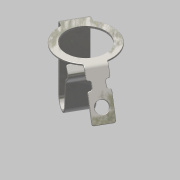
# Autodesk Inventor part: InputJack_signal2
Saved by Autodesk Inventor 2015 SP1 (Build 190203100, 203)
## iProperties
Created: 2015-06-13
Part Number: InputJack_signal2
Material: Generic
Document SubType Name: Modeling
Designer: Peter Mulkers
Density: 1 g/cm^3
Appearance: Titanium
Author: Peter Mulkers
Autodesk Inventor part; units mm, degrees
ref_plane "YZ Plane" through (0, 0, 0) normal (1, 0, 0) x (0, 1, 0)
ref_plane "XZ Plane" through (0, 0, 0) normal (0, 1, 0) x (-1, 0, 0)
ref_plane "XY Plane" through (0, 0, 0) normal (0, 0, 1) x (1, 0, 0)
sketch "Sketch1" plane through (0, 0, 0) normal (0, 0, 1) x (1, 0, 0)
  circle A0 centre (0, 0) radius 5.5
  line L0 (-6.9282, 4) -> (6.4952, -3.75) construction
  line L1 (0, 7.5) -> (0, -7.5) construction
  line L2 (-8.5532, 1.1854) -> (-5.3032, 6.8146)
  line L3 (-8.5532, 1.1854) -> (-7.4787, 0.565)
  line L4 (-5.3032, 6.8146) -> (-4.2287, 6.1942)
  line L5 (7.7452, -1.5849) -> (5.2452, -5.9151)
  line L6 (7.7452, -1.5849) -> (7.3737, -1.3705)
  line L7 (5.2452, -5.9151) -> (4.8737, -5.7006)
  arc A1 (-7.4787, 0.565) -> (4.8737, -5.7006) centre (0, 0) ccw
  arc A2 (7.3737, -1.3705) -> (-4.2287, 6.1942) centre (0, 0) ccw
  dimension "d0" = 11
  dimension "d2" = 60
  dimension "d3" = 6.5
  dimension "d4" = 8
  dimension "d5" = 15
  dimension "d6" = 5
  dimension "d7" = 7.5
  dimension "d8" = 7.5
  dimension "d9" = 7.5
  dimension "d10" = 2.5
  constraints: 16 end point, 7 point on circle, 4 perpendicular, 3 centre point, 3 midpoint, 2 coincident, 2 parallel, 1 point on line, 1 vertical alignment
  measures "d0" diameter of A0
  measures "d2" angle of L1 L0
  measures "d3" distance of L2.start L2.end
  measures "d4" distance from line of point (0, 0) L2
  measures "d5" distance of L1.start L1.end
  measures "d6" distance of L5.start L5.end
  measures "d7" radius of A2
  measures "d8" radius of A1
  measures "d9" distance from line of L5 A0.centre
  measures "d10" distance between parallel lines of L6 L0
extrude "Extrusion1" add sketch "Sketch1" along normal blind 0.5
sketch "Sketch2" plane through (5.6202, -6.1316, -0.25) normal (0.75, -0.4330127, 0.5) x (0.5, 0.8660254, 0)
  line L0 (5, 0) -> (0, 0)
  line L1 (0, 0) -> (0, -11.4226)
  line L2 (0, -11.4226) -> (5, -11.4226)
  line L3 (5, -11.4226) -> (5, 0)
  constraints: 8 end point
edge flange "Flange1" height 12 angle 60 thickness 0.5 bend radius 0.5 thickness toward (0.75, -0.4330127, 0.5) relief tear relief width 0.5 relief depth 0.25 edges at (6.4952, -3.75, 0) wall of the first edge with corners at (8.1202, -1.8014, -0.25) (5.6202, -6.1316, -0.25) (10.5663, -8.9872, -10.1423) (13.0663, -4.6571, -10.1423)
bend "Bend1"
corner "Corner1"
sketch "Sketch3" plane through (10.9413, -9.2037, -9.8923) normal (0.75, -0.4330127, 0.5) x (0.4330127, -0.25, -0.8660254)
  line L0 (-11.4226, 5) -> (-11.4226, 0) construction
  line L1 (0, 0) -> (-11.4226, 0) construction
  line L2 (0, 5) -> (0, 0) construction
  line L3 (-11.4226, 5) -> (0, 5) construction
  line L4 (-9, 0) -> (-9, 1)
  line L5 (-9, 1) -> (-7, 1)
  line L6 (-7, 1) -> (-7, 0)
  line L7 (-7, 0) -> (-9, 0)
  line L8 (-9, 5) -> (-9, 4)
  line L9 (-9, 4) -> (-7, 4)
  line L10 (-7, 4) -> (-7, 5)
  line L11 (-9, 5) -> (-7, 5)
  point P0 (-15.6057, 2.5)
  dimension "d23" = 1
  dimension "d25" = 2
  dimension "d26" = 7
  dimension "d27" = 1
  dimension "d28" = 2
  dimension "d29" = 7
  constraints: 16 end point, 4 perpendicular, 4 point on line, 2 collinear, 2 vertical
  measures "d23" distance between parallel lines of L5 L1
  measures "d25" distance between parallel lines of L6 L4
  measures "d26" distance between parallel lines of L2 L6
  measures "d27" distance between parallel lines of L3 L9
  measures "d28" distance between parallel lines of L10 L8
  measures "d29" distance between parallel lines of L2 L10
extrude "Extrusion2" cut sketch "Sketch3" against normal blind 0.5
fillet "Fillet1" radius 0.5 10 edges at (7.7228, -7.3455, -3.9551) (6.8567, -6.8455, -2.2231) (10.2228, -3.0154, -3.9551) (9.3567, -2.5154, -2.2231) (7.3567, -5.9795, -2.2231) (8.2228, -6.4795, -3.9551) (9.7228, -3.8814, -3.9551) (8.8567, -3.3814, -2.2231) (13.2538, -4.7654, -10.0173) (10.7538, -9.0955, -10.0173)
sketch "Sketch4" plane through (10.6268, -3.2486, -4.2631) normal (0.75, -0.4330127, 0.5) x (0.4330127, -0.25, -0.8660254)
  circle A0 centre (3, -2.5) radius 1.5
  line L0 (6.5, -0.5) -> (6.5, -4.5) projected
  point P0 (-9.1057, -2.5)
  point P1 (6.5, -2.5)
  dimension "d33" = 3
  dimension "d34" = 3.5
  constraints: 1 centre point, 1 horizontal alignment, 1 midpoint
  measures "d33" diameter of A0
  measures "d34" distance from line of A0.centre L0
extrude "Extrusion3" cut sketch "Sketch4" against normal blind 0.5
sketch "Sketch5" plane through (-5.7362, 7.0646, -0.5) normal (-0.8660254, 0.5, 0) x (-0.5, -0.8660254, 0)
  line L0 (6.5, 0) -> (0, 0)
  line L1 (0, 0) -> (0, -17)
  line L2 (0, -17) -> (6.5, -17)
  line L3 (6.5, -17) -> (6.5, 0)
  constraints: 6 end point, 1 horizontal, 1 perpendicular, 1 vertical
edge flange "Flange2" height 18 angle 90 thickness 0.5 bend radius 0.5 thickness toward (-0.8660254, 0.5, 0) relief tear relief width 0.5 relief depth 0.25 edges at (-6.9282, 4, 0) wall of the first edge with corners at (-8.9862, 1.4354, -0.5) (-5.7362, 7.0646, -0.5) (-5.7362, 7.0646, -17.5) (-8.9862, 1.4354, -17.5)
bend "Bend2"
corner "Corner2"
sketch "Sketch6" plane through (-9.4192, 1.6854, -17.5) normal (-0.5, -0.8660254, 0) x (0.8660254, -0.5, 0)
  line L0 (0, 17) -> (0, 0) construction
  arc A0 (0, 0) -> (4.9902, -0.2217) centre (2.5, 0) ccw
  line L1 (16.0711, 18) -> (2.2407, 18)
  line L2 (6, 10.5) -> (6, 7.5) construction
  line L3 (6, 9) -> (7.0607, 10.0607) construction
  line L4 (6, 9) -> (7.0607, 7.9393) construction
  line L5 (7.0607, 7.9393) -> (5.8421, 6.7208)
  line L6 (7.0607, 10.0607) -> (6, 11.1213)
  line L7 (4.9902, -0.2217) -> (5.5532, 6.1024)
  arc A1 (7.0607, 7.9393) -> (7.0607, 10.0607) centre (6, 9) ccw
  arc A2 (5.8421, 6.7208) -> (5.5532, 6.1024) centre (6.5492, 6.0137) ccw
  point P0 (9, 17.5)
  dimension "d47" = 5
  dimension "d48" = 9
  dimension "d50" = 6
  dimension "d51" = 45
  dimension "d52" = 45
  dimension "d53" = 1
  dimension "d54" = 1.5
  dimension "d55" = 1.5
  dimension "d56" = 1.7233
  dimension "d57" = 7.5
  dimension "d58" = 10.5
  measures "d47" diameter of A0
  measures "d48" distance from line of L1 L3.start
  measures "d50" distance from line of L0 L3.start
  measures "d51" angle of L3 L2
  measures "d52" angle of L4 L2
  measures "d53" radius of A2
  measures "d54" radius of A1
  measures "d55" distance of L3.end L6.end
  measures "d56" distance of L4.end L5.end
  measures "d57" distance from line of L2.start L1
  measures "d58" distance from line of L2.end L1
contour flange "Contour Flange1" sketch "Sketch6" thickness 0.5 bend radius 0.5 curves A0 L7 A2 L5 A1 L6 edges at (-7.3612, 4.25, -17.5) running between points at (-8.9862, 1.4354, -17.5) (-5.7362, 7.0646, -17.5)
bend "Bend3"
corner "Corner3"
fillet "Corner Round1" radius 0.5 6 edges at (-4.3762, -1.2262, -6.5555) (-1.1262, 4.403, -6.5555) (-7.4787, 0.565, 0.25) (-4.2287, 6.1942, 0.25) (4.8737, -5.7006, 0.25) (7.3737, -1.3705, 0.25)
fillet "Fillet2" radius 0.15 94 edges at (-7.5575, 0.528, 0.5) (-3.4091, -6.6804, 0.5) (4.8878, -5.8074, 0.5) (7.4733, -1.3293, 0.5) (4.0809, 6.2926, 0.5) (-4.236, 6.281, 0.5) (-9.1656, 1.539, 0.2071) (-9.4192, 1.6854, -9) (-7.3503, 0.4909, -19.9975) (-4.8538, -0.9504, -14.5597) (-4.532, -1.1362, -11.063) (-3.8322, -1.5403, -10.1699) (-2.924, -2.0646, -8.5) (-3.6107, -1.6681, -7.0858) (-4.0602, -1.2395, -6.4822) (-2.5981, 1.5, -6.3787) (-0.9566, 4.136, -6.4822) (-0.3607, 3.961, -7.0858) (0.326, 3.5646, -8.5) (-0.5822, 4.0889, -10.1699) (-1.282, 4.493, -11.063) (-1.6038, 4.6788, -14.5597) (-4.1003, 6.1201, -19.9975) (-6.1692, 7.3146, -9) (-5.9156, 7.1681, 0.2071) (8.1782, -1.8349, 0.366) (9.2942, -3.0566, -2.0981) (9.4076, -2.7138, -1.9713) (9.1808, -3.3994, -2.2249) (9.4772, -3.7396, -2.9641) (10.1603, -3.5566, -3.8301) (9.9201, -3.8262, -3.7033) (10.4004, -3.287, -3.9569) (11.9258, -3.9986, -6.8612) (13.3047, -4.9638, -9.7655) (12.1913, -7.0387, -9.8923) (10.9512, -9.0403, -9.7655) (9.4258, -8.3287, -6.8612) (8.0469, -7.3635, -3.9569) (8.1603, -7.0207, -3.8301) (8.2736, -6.6779, -3.7033) (7.9772, -6.3377, -2.9641) (7.5344, -6.2511, -2.2249) (7.2942, -6.5207, -2.0981) (7.054, -6.7903, -1.9713) (5.6782, -6.1651, 0.366) (-4.1383, -1.3635, -9.8164) (-4.9243, -0.9097, -10.8513) (-5.2851, -0.7014, -14.5153) (-7.331, 0.4798, -19.498) (-8.9862, 1.4354, -9) (-8.8594, 1.3622, -0.1464) (-7.5575, 0.528, 0) (-3.4091, -6.6804, 0) (4.8878, -5.8074, 0) (5.4617, -6.0401, -0.067) (6.679, -6.5738, -2.2213) (6.9192, -6.3042, -2.3481) (7.1594, -6.0346, -2.4749) (7.6022, -6.1212, -3.2141) (7.8986, -6.4614, -3.9533) (7.7853, -6.8042, -4.0801) (7.6719, -7.147, -4.2069) (9.0508, -8.1122, -7.1112) (10.5762, -8.8238, -10.0155) (11.8163, -6.8222, -10.1423) (12.9297, -4.7473, -10.0155) (11.5508, -3.7821, -7.1112) (9.7853, -3.3401, -4.0801) (10.0254, -3.0705, -4.2069) (9.5451, -3.6097, -3.9533) (9.1022, -3.5231, -3.2141) (8.9192, -2.8401, -2.3481) (8.8058, -3.1829, -2.4749) (9.0326, -2.4973, -2.2213) (7.9617, -1.7099, -0.067) (7.4733, -1.3293, 0) (4.0809, 6.2926, 0) (-4.236, 6.281, 0) (-5.6094, 6.9914, -0.1464) (-5.7362, 7.0646, -9) (-4.081, 6.109, -19.498) (-2.0351, 4.9278, -14.5153) (-1.6743, 4.7195, -10.8513) (-0.8883, 4.2657, -9.8164) (-0.1071, 3.8146, -8.5) (-0.6669, 4.1378, -7.4393) (-1.2628, 4.3128, -6.8358) (-2.9043, 1.6768, -6.7322) (-4.3664, -1.0628, -6.8358) (-3.9169, -1.4914, -7.4393) (-3.3571, -1.8146, -8.5) (10.0263, -5.7887, -5.5622) (9.6513, -5.5722, -5.8122)
equation "\"d13\" = BendReliefWidth"
equation "\"d14\" = BendReliefDepth"
equation "\"d15\" = MinimumRemnant"
equation "\"d16\" = BendRadius"
equation "\"d19\" = BendRadius"
equation "\"d20\" = CornerReliefSize"
equation "\"d21\" = GapSize"
equation "\"d22\" = JacobiRadiusSize"
equation "\"d37\" = BendReliefWidth"
equation "\"d38\" = BendReliefDepth"
equation "\"d39\" = MinimumRemnant"
equation "\"d40\" = BendRadius"
equation "\"d43\" = BendRadius"
equation "\"d44\" = CornerReliefSize"
equation "\"d45\" = GapSize"
equation "\"d46\" = JacobiRadiusSize"
equation "\"d59\" = BendReliefWidth"
equation "\"d60\" = BendReliefDepth"
equation "\"d61\" = MinimumRemnant"
equation "\"d62\" = BendRadius"
equation "\"d63\" = BendRadius"
equation "\"d65\" = CornerReliefSize"
equation "\"d66\" = GapSize"
equation "\"d67\" = JacobiRadiusSize"
equation "\"BendRadius\" = Thickness"
equation "\"BendReliefWidth\" = Thickness"
equation "\"BendReliefDepth\" = 0.5 * Thickness"
equation "\"CornerReliefSize\" = 4 * Thickness"
equation "\"MinimumRemnant\" = 2 * Thickness"
equation "\"TransitionRadius\" = BendRadius"
equation "\"JacobiRadiusSize\" = BendRadius"
equation "\"GapSize\" = Thickness"
equation "\"Thickness\" = 0.5"
body "Solid1"
